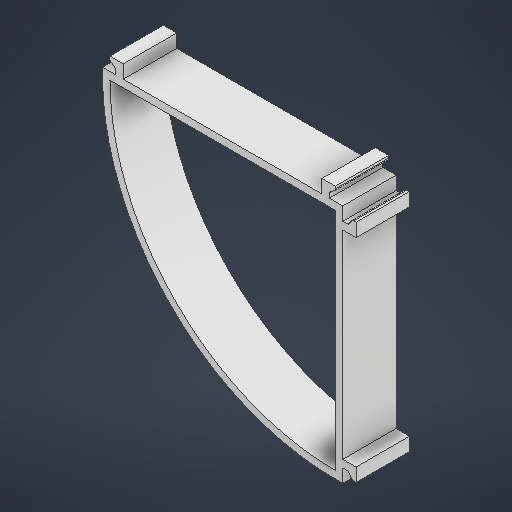
# Autodesk Inventor part: SP40-15 PERFIL ESQUINERO PUNTAS INVERTIDAS
Saved by Autodesk Inventor 2025 (Build 290162000, 162)
## iProperties
Created: 2026-01-30
Part Number: SP40-15 PERFIL ESQUINERO PUNTAS INVERTIDAS
Material: Aluminio
Document SubType Name: Modeling
Designer: ROLANDO
Density: 2.7 g/cm^3
Appearance: Satinado
Author: ROLANDO
Autodesk Inventor part; units mm, degrees
ref_plane "YZ Plane" through (0, 0, 0) normal (1, 0, 0) x (0, 1, 0)
ref_plane "XZ Plane" through (0, 0, 0) normal (0, 1, 0) x (-1, 0, 0)
ref_plane "XY Plane" through (0, 0, 0) normal (0, 0, 1) x (1, 0, 0)
sketch "Boceto1" plane through (0, 0, 0) normal (0, 0, 1) x (1, 0, 0)
  line L0 (43.6, -1.4) -> (1.4, -1.4)
  line L1 (0, -1.4) -> (0, 0)
  line L2 (45, -45) -> (43.6, -45)
  line L3 (43.6, -43.6) -> (43.6, -1.4)
  arc A0 (1.4, -1.4) -> (43.6, -43.6) centre (43.6, -1.4) ccw
  arc A1 (0, -1.4) -> (43.6, -45) centre (43.6, -1.4) ccw
  line L4 (2.5, 0) -> (2.5, 0.7532)
  line L5 (2.2918, 1.1592) -> (1.4, 1.8)
  line L6 (1.4, 1.8) -> (1.4, 2.5)
  line L7 (1.4, 2.5) -> (3.9, 2.5)
  line L8 (3.9, 2.5) -> (3.9, 0)
  arc A2 (2.5, 0.7532) -> (2.2918, 1.1592) centre (2, 0.7532) ccw
  line L9 (0, 0) -> (2.5, 0)
  line L10 (42.5, 0) -> (42.5, 0.8223)
  line L11 (42.7447, 1.2522) -> (43.3553, 1.6147)
  line L12 (43.6, 2.0446) -> (43.6, 2.5)
  line L13 (43.6, 2.5) -> (41.1, 2.5)
  line L14 (41.1, 2.5) -> (41.1, 0)
  line L15 (3.9, 0) -> (41.1, 0)
  line L16 (42.5, 0) -> (45, 0)
  arc A3 (42.7447, 1.2522) -> (42.5, 0.8223) centre (43, 0.8223) ccw
  arc A4 (43.3553, 1.6147) -> (43.6, 2.0446) centre (43.1, 2.0446) ccw
  line L17 (45, -2.5) -> (45.8223, -2.5)
  line L18 (46.2522, -2.2553) -> (46.6147, -1.6447)
  line L19 (47.0446, -1.4) -> (47.5, -1.4)
  line L20 (47.5, -1.4) -> (47.5, -3.9)
  line L21 (47.5, -3.9) -> (45, -3.9)
  arc A5 (47.0446, -1.4) -> (46.6147, -1.6447) centre (47.0446, -1.9) ccw
  arc A6 (45.8223, -2.5) -> (46.2522, -2.2553) centre (45.8223, -2) ccw
  line L22 (45, -42.5) -> (45.7532, -42.5)
  line L23 (46.1592, -42.7082) -> (46.8, -43.6)
  line L24 (46.8, -43.6) -> (47.5, -43.6)
  line L25 (47.5, -43.6) -> (47.5, -41.1)
  line L26 (47.5, -41.1) -> (45, -41.1)
  arc A7 (46.1592, -42.7082) -> (45.7532, -42.5) centre (45.7532, -43) ccw
  line L27 (45, -0.1052) -> (45, -2.5)
  line L28 (45, -2.5) -> (45, 0)
  line L29 (45, -3.9) -> (45, -41.1)
  line L30 (45, -42.5) -> (45, -45)
  line L31 (45, -45) -> (45, -42.5)
  line L32 (45, -41.1) -> (45, -3.9)
  point P0 (43.6, 1.76)
  point P1 (46.76, -1.4)
  dimension "d11" = 42.2
  dimension "d12" = 1.4
  dimension "d18" = 1.4
  dimension "d19" = 2.5
  dimension "d21" = 2.5
  dimension "d25" = 35.7
  dimension "d26" = 1.4
  dimension "d28" = 1.4
  dimension "d29" = 0.74
  dimension "d30" = 2.5
  dimension "d31" = 30.7
  dimension "d32" = 2.5
  dimension "d34" = 0.5
  dimension "d35" = 0.7
  dimension "d36" = 0.5
  dimension "d37" = 0.5
  dimension "d38" = 1.4
  dimension "d39" = 2.5
  dimension "d41" = 2.5
  dimension "d42" = 0.74
  dimension "d43" = 30.7
  dimension "d44" = 0.5
  dimension "d45" = 45
  dimension "d46" = 1.4
  dimension "d47" = 2.5
  dimension "d49" = 0.7
  dimension "d50" = 35.7
  dimension "d51" = 2.5
  dimension "d52" = 0.5
  dimension "d55" = 1.4
  dimension "d57" = 2.5
  dimension "d58" = 45
  dimension "d59" = 2.5
  dimension "d63" = 2.5
  dimension "d64" = 2.5
  constraints: 66 end point, 32 perpendicular, 16 point on circle, 12 tangent, 8 centre point, 6 collinear, 5 coincident, 5 vertical, 4 horizontal, 4 parallel, 4 point on line, 1 equal radius, 2 other
  measures "d11" radius of A0
  measures "d12" radial gap between concentric circles of A0 A1
  measures "d18" distance between parallel lines of L4 L8
  measures "d19" distance from line of point (0, 0) L4
  measures "d21" distance of L6.end L7.end
  measures "d25" angle of L7 L5
  measures "d26" distance between parallel lines of L14 L10
  measures "d28" distance between parallel lines of L15 L0
  measures "d29" distance of point (43.6, 1.76) L12.end
  measures "d30" distance of L12.end L13.end
  measures "d31" angle of L13 L11
  measures "d32" distance between parallel lines of L15 L13
  measures "d34" radius of A3
  measures "d35" distance of L5.end L6.end
  measures "d36" radius of A4
  measures "d37" radius of A2
  measures "d38" distance between parallel lines of L21 L17
  measures "d39" distance from line of L17 L16.end
  measures "d41" distance of L19.end L20.end
  measures "d42" distance of point (46.76, -1.4) L19.end
  measures "d43" angle of L18 L20
  measures "d44" radius of A5
  measures "d45" distance between parallel lines of L2 L15
  measures "d46" distance between parallel lines of L26 L22
  measures "d47" distance from line of L30.end L22
  measures "d49" distance of L23.end L24.end
  measures "d50" angle of L25 L23
  measures "d51" distance of L24.end L25.end
  measures "d52" radius of A7
  measures "d55" distance between parallel lines of L3 L29
  measures "d57" distance between parallel lines of L29 L20
  measures "d58" distance between parallel lines of L29 L1
  measures "d59" distance from line of L16.end L10
  measures "d63" distance of L25.end L26.end
  measures "d64" distance of L7.end L8.end
extrude "Extrusión1" add sketch "Boceto1" against normal blind 10
